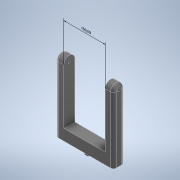
# Autodesk Inventor part: AERO - Fork
Saved by Autodesk Inventor 2021 (Build 250183000, 183)
## iProperties
Created: 2021-01-21
Part Number: AERO - Fork
Material: Generic
Document SubType Name: Modeling
Designer: garciar1
Density: 1 g/cm^3
Appearance: Smooth - Black
Author: garciar1
Autodesk Inventor part; units mm, degrees
ref_plane "YZ Plane" through (0, 0, 0) normal (1, 0, 0) x (0, 1, 0)
ref_plane "XZ Plane" through (0, 0, 0) normal (0, 1, 0) x (-1, 0, 0)
ref_plane "XY Plane" through (0, 0, 0) normal (0, 0, 1) x (1, 0, 0)
sketch "Sketch1" plane through (0, 0, 0) normal (1, 0, 0) x (0, 1, 0)
  line L0 (0, 20) -> (40, 20)
  line L1 (40, 20) -> (40, -20)
  line L2 (40, -20) -> (0, -20)
  line L3 (0, -20) -> (0, 20)
  point P0 (0, 0)
  dimension "d0" = 20
  dimension "d1" = 40
  dimension "d2" = 40
  dimension "d3" = 40
  constraints: 8 end point, 2 parallel, 1 horizontal, 1 perpendicular
  measures "d0" distance from line of L0 point (0, 0)
  measures "d1" distance of L1.end L2.end
  measures "d2" distance of L0.end L1.end
  measures "d3" distance from line of L1 point (0, 0)
extrude "Extrusion1" add sketch "Sketch1" along normal mid plane 210
sketch "Sketch2" plane through (-105, 40, 20) normal (0, 1, 0) x (1, 0, 0)
  line L0 (210, 40) -> (210, 0) projected
  line L1 (0, 40) -> (210, 40) projected
  line L2 (210, 0) -> (180, 0)
  line L3 (180, 0) -> (180, 40)
  line L4 (180, 40) -> (210, 40)
  line L5 (210, 40) -> (210, 0)
  line L6 (0, 0) -> (210, 0) projected
  line L7 (0, 0) -> (30, 0)
  line L8 (30, 0) -> (30, 40)
  line L9 (30, 40) -> (0, 40)
  line L10 (0, 40) -> (0, 0)
  point P0 (105, 20)
  point P1 (0, 40)
  point P2 (30, 0)
  point P3 (30, 40)
  dimension "d6" = 30
  dimension "d7" = 30
  constraints: 16 end point, 4 parallel, 2 horizontal, 2 perpendicular, 2 point on line
  measures "d6" distance between parallel lines of L10 L8
  measures "d7" distance between parallel lines of L0 L3
extrude "Extrusion2" add sketch "Sketch2" along normal blind 200 contours L0 L2 L3 L1 | L8 L6 L10 L1
sketch "Sketch3" plane through (-75, 40, 20) normal (1, 0, 0) x (0, 0, -1)
  line L0 (40, 200) -> (0, 200) projected
  circle A0 centre (20, 200) radius 20
  circle A1 centre (20, 200) radius 5
  point P0 (20, -40)
  dimension "d14" = 10
  constraints: 1 centre point, 1 coincident, 1 horizontal alignment, 1 midpoint, 2 other
  measures "d14" diameter of A1
extrude "Extrusion3" add sketch "Sketch3" against normal up to surface (30 mm away)
sketch "Sketch4" plane through (105, 0, 0) normal (1, 0, 0) x (0, 0, -1)
  arc A0 (20, 240) -> (-20, 240) centre (0, 240) ccw projected
  line L0 (-20, 240) -> (20, 240) projected
  circle A1 centre (0, 240) radius 20
  point P0 (0, 0)
  point P1 (-20, 240)
  constraints: 1 coincident, 3 other
extrude "Extrusion4" add sketch "Sketch4" against normal up to surface (30 mm away)
sketch "Sketch5" plane through (105, 0, 0) normal (1, 0, 0) x (0, 0, -1)
  arc A0 (20, 240) -> (-20, 240) centre (0, 240) ccw projected
  circle A1 centre (0, 240) radius 5
  point P0 (0, 0)
  dimension "d15" = 10
  constraints: 1 centre point, 1 coincident
  measures "d15" diameter of A1
extrude "Extrusion5" cut sketch "Sketch5" against normal through all
fillet "Fillet1" radius 10 6 edges at (105, 120, 20) (105, 120, -20) (105, 260, 0) (-105, 120, -20) (-105, 120, 20) (-105, 260, 0)
sketch "Sketch6" plane through (-95, 0, -20) normal (0, -1, 0) x (1, 0, 0)
  circle A0 centre (95, 20) radius 15
  dimension "d21" = 30
  constraints: 1 centre point, 1 coincident
  measures "d21" diameter of A0
extrude "Extrusion6" add sketch "Sketch6" along normal blind 10
body "Solid1"
